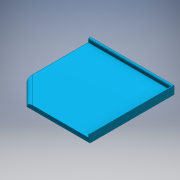
# Autodesk Inventor part: meson_esquinero
Saved by Autodesk Inventor 2016 (Build 200138000, 138)
## iProperties
Created: 2015-11-25
Part Number: meson_esquinero
Material: Generic
Document SubType Name: Modeling
Designer: Daniela
Density: 1 g/cm^3
Appearance: Exposed Aggregate - Warm Gray
Author: Daniela
Autodesk Inventor part; units mm, degrees
ref_plane "YZ Plane" through (0, 0, 0) normal (1, 0, 0) x (0, 1, 0)
ref_plane "XZ Plane" through (0, 0, 0) normal (0, 1, 0) x (-1, 0, 0)
ref_plane "XY Plane" through (0, 0, 0) normal (0, 0, 1) x (1, 0, 0)
sketch "Sketch1" plane through (0, 0, 0) normal (0, 0, 1) x (1, 0, 0)
  line L0 (0, 0) -> (1050, 0) construction
  line L1 (1050, 0) -> (1050, 1050)
  line L2 (1050, 1050) -> (0, 1050)
  line L3 (0, 1050) -> (0, 0) construction
  line L4 (0, 260) -> (260, 0)
  line L5 (0, 260) -> (0, 1050)
  line L6 (260, 0) -> (1050, 0)
  dimension "profundidad" = 790
  dimension "d22" = 790
  dimension "d23" = 1050
  constraints: 14 end point, 2 collinear, 2 parallel, 2 perpendicular, 2 point on line, 1 horizontal
  measures "profundidad" distance of L4.start L2.end
  measures "d22" distance of L0.end L4.end
  measures "d23" distance of L1.end L2.end
extrude "Extrusion1" add sketch "Sketch1" along normal blind 50
fillet "Fillet1" radius 50 1 edges at (130, 130, 50)
sketch "Sketch3" plane through (1050, 0, 0) normal (0, -1, 0) x (1, 0, 0)
  line L0 (-1050, 0) -> (0, 0) projected
  line L1 (0, 0) -> (-20, 0)
  line L2 (-20, 0) -> (-20, 80)
  line L3 (0, 100) -> (0, 100)
  line L4 (0, 100) -> (0, 0)
  arc A0 (0, 100) -> (-20, 80) centre (0, 80) ccw
  point P0 (-20, 100)
  dimension "d9" = 20
  dimension "d10" = 100
  dimension "d11" = 20
  constraints: 8 end point, 2 parallel, 2 point on circle, 2 point on line, 2 tangent, 1 centre point, 1 horizontal, 1 perpendicular
  measures "d9" distance of point (-20, 100) L3.end
  measures "d10" distance of L1.end point (-20, 100)
  measures "d11" radius of A0
extrude "Extrusion2" add sketch "Sketch3" against normal up to surface (1050 mm away)
sketch "Sketch4" plane through (0, 1050, 0) normal (-1, 0, 0) x (0, 0, 1)
  line L0 (0, 0) -> (100, 0) projected
  line L1 (100, -1050) -> (100, 0) projected
  line L2 (0, 0) -> (100, 0)
  line L3 (100, 0) -> (100, 0)
  line L4 (80, -20) -> (0, -20)
  line L5 (0, -20) -> (0, 0)
  arc A0 (80, -20) -> (100, 0) centre (80, 0) ccw
  point P0 (0, -1050)
  point P1 (100, -20)
  dimension "d14" = 20
  dimension "d15" = 20
  constraints: 8 end point, 3 point on line, 2 parallel, 2 point on circle, 2 tangent, 1 centre point, 1 horizontal, 1 perpendicular
  measures "d14" distance between parallel lines of L0 L4
  measures "d15" radius of A0
extrude "Extrusion3" add sketch "Sketch4" against normal up to surface (1050 mm away)
body "Solid1"
